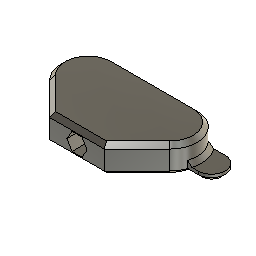
5mm_Hex_Key (Autodesk Fusion 360 design; units mm, degrees)
Autodesk Fusion 360 part; units mm, degrees
sketch "Sketch1" plane through (0, 0, 0) normal (0, 0, 1) x (1, 0, 0)
  line L0 (-10, 0) -> (10, 0)
  line L1 (10, 0) -> (22.0711, 12.0711)
  arc A0 (22.0711, 12.0711) -> (15, 29.1421) centre (15, 19.1421) ccw
  line L2 (15, 29.1421) -> (-15, 29.1421)
  arc A1 (-15, 29.1421) -> (-22.0711, 12.0711) centre (-15, 19.1421) ccw
  line L3 (-22.0711, 12.0711) -> (-10, 0)
  line L4 (0, 0) -> (0, 29.1421) construction
  line L5 (-24, 23.501) -> (-24, 41.501)
  line L6 (-24, 41.501) -> (-18, 41.501)
  line L7 (-18, 41.501) -> (-18, 28.6815)
  line L8 (22.1414, 26.1421) -> (28.351, 26.1421)
  arc A2 (28.351, 16.1421) -> (28.351, 26.1421) centre (28.351, 21.1421) ccw
  line L9 (28.351, 16.1421) -> (24.5394, 16.1421)
  dimension "d1" = 10
  dimension "d2" = 135
  dimension "d3" = 50
  dimension "d4" = 20
  dimension "d5" = 6
  dimension "d6" = 18
  dimension "d7" = 18
  dimension "d18" = 5
  dimension "d19" = 3
  dimension "d20" = 3.5
  constraint horizontal L0
  constraint tangent L1 A0
  constraint parallel L0 L2
  constraint tangent L2 A1
  constraint tangent A1 L3
  constraint tangent A0 L2
  constraint midpoint L0 L4.start
  constraint midpoint L2 L4.end
  constraint vertical L4
  constraint coincident L4.start origin
  constraint perpendicular L1 L3
  constraint coincident A1 L5.start
  constraint vertical L5
  constraint perpendicular L5 L6
  constraint perpendicular L2 L7
  constraint coincident A1 L7.end
  constraint coincident A0 L8.start
  constraint horizontal L8
  constraint tangent L8 A2
  constraint tangent A2 L9
  constraint coincident A0 L9.end
  constraint horizontal L9
  measures "d1" radius of A1
  measures "d2" angle of L0 L1
  measures "d4" distance of L0.start L0.end
  measures "d5" distance of L5.end L6.end
  measures "d6" distance of L5.start L5.end
  measures "d7" horizontal distance of L4.start L7.end
  measures "d18" radius of A2
  measures "d19" distance of L2 L8
  measures "d20" distance of A0 A2.centre
extrude "Extrude1" add sketch "Sketch1" along normal mid plane 10 contours L0 L1 A0 L2 A1 L3
extrude "Extrude3" add sketch "Sketch1" along normal blind 2.6 from surface at -5 contours A0 L8 A2 L9
sketch "Sketch2" plane through (0, 0, 0) normal (0, 1, 0) x (1, 0, 0)
  line L0 (3.695, 0) -> (1.8475, 3.2)
  line L1 (1.8475, 3.2) -> (-1.8475, 3.2)
  line L2 (-1.8475, 3.2) -> (-3.695, 0)
  line L3 (-3.695, 0) -> (-1.8475, -3.2)
  line L4 (-1.8475, -3.2) -> (1.8475, -3.2)
  line L5 (1.8475, -3.2) -> (3.695, 0)
  dimension "d10" = 6.4
  constraint horizontal L4
  measures "d10" distance of L0.end L4.end
extrude "Extrude2" cut sketch "Sketch2" along normal blind 16
chamfer "Chamfer1" distance 1.5 angle 45 1 edges at (24.7243, 21.474, -2.4) 2 faces at (3.3333, 19.4281, 5) (3.3333, 19.4281, -5)
